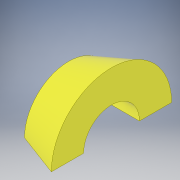
# Autodesk Inventor part: parachute
Saved by Autodesk Inventor 2019.3 (Build 233278000, 278)
## iProperties
Created: 2019-01-10
Part Number: parachute
Material: 一般
Document SubType Name: Modeling
Designer: masaya
Density: 1 g/cm^3
Appearance: 滑らか - 黄
Author: masaya
Autodesk Inventor part; units mm, degrees
ref_plane "YZ Plane" through (0, 0, 0) normal (1, 0, 0) x (0, 1, 0)
ref_plane "XZ Plane" through (0, 0, 0) normal (0, 1, 0) x (-1, 0, 0)
ref_plane "XY Plane" through (0, 0, 0) normal (0, 0, 1) x (1, 0, 0)
sketch "スケッチ1" plane through (0, 0, 0) normal (0, 1, 0) x (-1, 0, 0)
  line L0 (0, 130) -> (0, 280)
  line L1 (0, 280) -> (200, 204.9843)
  line L2 (200, 204.9843) -> (200, 130)
  line L3 (200, 130) -> (0, 130)
  line L4 (240, 0) -> (-40, 0) projected
  line L5 (0, -56) -> (0, 336) projected
  point P0 (0, 0)
  dimension "d0" = 150
  dimension "d1" = 69.44
  dimension "d2" = 200
  dimension "d3" = 130
  constraints: 8 end point, 2 vertical, 1 collinear, 1 perpendicular
  measures "d0" distance of L0.start L0.end
  measures "d1" angle of L0 L1
  measures "d2" distance of L2.end L0.start
  measures "d3" distance between parallel lines of L4 L3
revolve "回転1" add sketch "スケッチ1" angle 180 about axis through (-10, 0, 0) along (-1, 0, 0)
